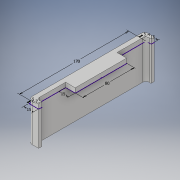
# Autodesk Inventor part: Part2
Saved by Autodesk Inventor 2018 (Build 220112000, 112)
## iProperties
Created: 2019-02-25
Part Number: Part2
Material: Generic
Document SubType Name: Modeling
Designer: ayoub
Density: 1 g/cm^3
Appearance: Default
Author: ayoub
Autodesk Inventor part; units mm, degrees
(part 1 of 2)
ref_plane "YZ Plane" through (0, 0, 0) normal (1, 0, 0) x (0, 1, 0)
ref_plane "XZ Plane" through (0, 0, 0) normal (0, 1, 0) x (-1, 0, 0)
ref_plane "XY Plane" through (0, 0, 0) normal (0, 0, 1) x (1, 0, 0)
sketch "Sketch1" plane through (0, 0, 0) normal (0, 1, 0) x (-1, 0, 0)
  line L0 (0, 40) -> (15, 40)
  line L1 (15, 40) -> (15, -40)
  line L2 (15, -40) -> (0, -40)
  line L3 (0, -40) -> (0, 40)
  line L4 (15, 85) -> (22, 85)
  line L5 (22, 85) -> (22, -85)
  line L6 (22, -85) -> (15, -85)
  line L7 (15, -85) -> (15, 85)
  line L8 (22, 85) -> (7, 85)
  line L9 (7, 85) -> (7, 90)
  line L10 (7, 90) -> (22, 90)
  line L11 (22, 90) -> (22, 85)
  line L12 (22, -85) -> (7, -85)
  line L13 (7, -85) -> (7, -90)
  line L14 (7, -90) -> (22, -90)
  line L15 (22, -90) -> (22, -85)
  point P0 (0, 0)
  point P1 (0, 0)
  point P2 (15, 0)
  dimension "d0" = 80
  dimension "d1" = 15
  dimension "d4" = 15
  dimension "d5" = 15
  dimension "d6" = 5
  dimension "d7" = 170
  dimension "d8" = 5
  dimension "d9" = 7
  constraints: 32 end point, 8 parallel, 4 horizontal, 4 perpendicular, 3 midpoint, 1 coincident
  measures "d0" distance of L2.end L0.start
  measures "d1" distance of L0.start L0.end
  measures "d4" distance of L9.end L10.end
  measures "d5" distance of L13.end L14.end
  measures "d6" distance of L10.end L4.end
  measures "d7" distance of L6.end L4.start
  measures "d8" distance of L14.end L5.end
  measures "d9" distance of L4.start L4.end
extrude "Extrusion1" add sketch "Sketch1" along normal blind 7 contours L0 L1 L2 L3
extrude "Extrusion2" add sketch "Sketch1" along normal blind 7 and the other way blind 53 contours L7 L4 L5 L6 L1
extrude "Extrusion3" add sketch "Sketch1" along normal blind 7 and the other way blind 53 contours L8 L9 L10 L11 L4 | L6 L15 L14 L13 L12
fillet "Fillet1" radius 5 1 edges at (-22, -23, 90)
fillet "Fillet2" radius 5 1 edges at (-22, -23, -90)
fillet "Fillet3" radius 5 1 edges at (-15, -23, -85)
fillet "Fillet4" radius 5 1 edges at (-15, -23, 85)
sketch "Sketch2" plane through (-22, -53, 85) normal (-1, 0, 0) x (0, 0, 1)
  line L0 (-170, 0) -> (-170, 60) projected
  line L1 (-18, 7.3167) -> (-152, 7.3167) construction
  line L2 (-152, 7.3167) -> (-152, 22.3167) construction
  line L3 (-152, 27.3167) -> (-18, 27.3167) construction
  line L4 (-18, 27.3167) -> (-18, 7.3167) construction
  line L5 (0, 60) -> (0, 0) projected
  line L6 (-147, 7.3167) -> (-142, 7.3167)
  line L7 (-142, 7.3167) -> (-142, 12.3167)
  line L8 (-142, 12.3167) -> (-146, 12.3167)
  line L9 (-147, 13.3167) -> (-147, 21.3167)
  line L10 (-146, 22.3167) -> (-142, 22.3167)
  line L11 (-142, 22.3167) -> (-142, 27.3167)
  line L12 (-142, 27.3167) -> (-147, 27.3167)
  line L13 (-28, 7.3167) -> (-23, 7.3167)
  line L14 (-23, 27.3167) -> (-28, 27.3167)
  line L15 (-28, 27.3167) -> (-28, 22.3167)
  line L16 (-28, 12.3167) -> (-28, 7.3167)
  line L17 (-18, 12.3167) -> (-18, 22.3167)
  arc A0 (-23, 7.3167) -> (-18, 12.3167) centre (-23, 12.3167) ccw
  arc A1 (-18, 22.3167) -> (-23, 27.3167) centre (-23, 22.3167) ccw
  arc A2 (-147, 27.3167) -> (-152, 22.3167) centre (-147, 22.3167) ccw
  arc A3 (-152, 12.3167) -> (-147, 7.3167) centre (-147, 12.3167) ccw
  arc A4 (-147, 13.3167) -> (-146, 12.3167) centre (-146, 13.3167) ccw
  arc A5 (-146, 22.3167) -> (-147, 21.3167) centre (-146, 21.3167) ccw
  line L18 (-51.6825, 53.4391) -> (-114.3216, 53.4391) construction
  line L19 (-114.3216, 53.4391) -> (-114.3216, 31.9963) construction
  line L20 (-114.3216, 31.9963) -> (-51.6825, 31.9963) construction
  line L21 (-51.6825, 31.9963) -> (-51.6825, 53.4391) construction
  line L22 (-152, 12.3167) -> (-152, 22.3167)
  line L23 (-24, 12.3167) -> (-28, 12.3167)
  line L24 (-24, 22.3167) -> (-28, 22.3167)
  line L25 (-23, 13.3167) -> (-23, 21.3167)
  arc A6 (-24, 12.3167) -> (-23, 13.3167) centre (-24, 13.3167) ccw
  arc A7 (-23, 21.3167) -> (-24, 22.3167) centre (-24, 21.3167) ccw
  line L26 (-147.3155, 50.9956) -> (-166.2914, 50.9956) construction
  line L27 (-166.2914, 50.9956) -> (-166.2914, 58.7345) construction
  line L28 (-166.2914, 58.7345) -> (-147.3155, 58.7345) construction
  line L29 (-147.3155, 58.7345) -> (-147.3155, 50.9956) construction
  line L30 (-48.6554, 17.8276) -> (-37.2597, 17.8276)
  spline S0 degree 2 poles (-37.2597, 17.8276) (-37.3507, 18.212) (-39.1918, 18.6925) (-40.4209, 18.6925) knots 0 0 0 1 2 2 2
  spline S1 degree 2 poles (-40.4209, 18.6925) (-42.6111, 18.6925) (-43.8553, 18.1968) knots 0 0 0 1 1 1
  line L31 (-43.8553, 18.1968) -> (-48.2255, 18.561)
  spline S2 degree 2 poles (-48.2255, 18.561) (-45.7926, 19.6232) (-40.6637, 19.6232) knots 0 0 0 1 1 1
  spline S3 degree 2 poles (-40.6637, 19.6232) (-36.8904, 19.6232) (-32.4292, 18.4801) (-32.4292, 17.514) knots 0 0 0 1 2 2 2
  spline S4 degree 2 poles (-32.4292, 17.514) (-32.4292, 16.644) (-37.1332, 15.4655) (-40.5727, 15.4655) knots 0 0 0 1 2 2 2
  spline S5 degree 2 poles (-40.5727, 15.4655) (-44.0273, 15.4655) (-48.6554, 16.7047) (-48.6554, 17.6354) knots 0 0 0 1 2 2 2
  line L32 (-48.6554, 17.6354) -> (-48.6554, 17.8276)
  line L33 (-37.2951, 17.0284) -> (-43.7289, 17.0284)
  spline S6 degree 2 poles (-43.7289, 17.0284) (-43.0612, 16.2798) (-40.6587, 16.2798) knots 0 0 0 1 1 1
  spline S7 degree 2 poles (-40.6587, 16.2798) (-39.2829, 16.2798) (-37.4822, 16.6693) (-37.2951, 17.0284) knots 0 0 0 1 2 2 2
  line L34 (-50.7393, 15.5414) -> (-56.5763, 15.5414)
  line L35 (-56.5763, 15.5414) -> (-59.8084, 16.5378)
  line L36 (-59.8084, 16.5378) -> (-63.0051, 15.5414)
  line L37 (-63.0051, 15.5414) -> (-68.8269, 15.5414)
  line L38 (-68.8269, 15.5414) -> (-62.7117, 17.4533)
  line L39 (-62.7117, 17.4533) -> (-69.4035, 19.5372)
  line L40 (-69.4035, 19.5372) -> (-63.5311, 19.5372)
  line L41 (-63.5311, 19.5372) -> (-59.8034, 18.3587)
  line L42 (-59.8034, 18.3587) -> (-56.0402, 19.5372)
  line L43 (-56.0402, 19.5372) -> (-50.183, 19.5372)
  line L44 (-50.183, 19.5372) -> (-56.8495, 17.4482)
  line L45 (-56.8495, 17.4482) -> (-50.7393, 15.5414)
  line L46 (-77.0715, 15.5515) -> (-77.0715, 16.1332)
  line L47 (-77.0715, 16.1332) -> (-77.1474, 16.1332)
  spline S8 degree 2 poles (-77.1474, 16.1332) (-78.1893, 15.7841) (-80.4351, 15.4655) (-82.0183, 15.4655) knots 0 0 0 1 2 2 2
  spline S9 degree 2 poles (-82.0183, 15.4655) (-84.8811, 15.4655) (-88.9175, 16.7199) (-88.9175, 17.6152) knots 0 0 0 1 2 2 2
  spline S10 degree 2 poles (-88.9175, 17.6152) (-88.9175, 18.4396) (-84.9924, 19.6131) (-82.2965, 19.6131) knots 0 0 0 1 2 2 2
  spline S11 degree 2 poles (-82.2965, 19.6131) (-80.6425, 19.6131) (-78.4119, 19.2691) (-77.2233, 18.8948) knots 0 0 0 1 2 2 2
  line L48 (-77.2233, 18.8948) -> (-77.1474, 18.8948)
  line L49 (-77.1474, 18.8948) -> (-77.1474, 21.2974)
  line L50 (-77.1474, 21.2974) -> (-72.317, 21.2974)
  line L51 (-72.317, 21.2974) -> (-72.317, 15.5515)
  line L52 (-72.317, 15.5515) -> (-77.0715, 15.5515)
  spline S12 degree 2 poles (-83.9353, 17.605) (-83.9353, 17.2156) (-81.9272, 16.6541) (-80.5312, 16.6541) knots 0 0 0 1 2 2 2
  spline S13 degree 2 poles (-80.5312, 16.6541) (-79.1554, 16.6541) (-77.2233, 17.2055) (-77.2233, 17.605) knots 0 0 0 1 2 2 2
  spline S14 degree 2 poles (-77.2233, 17.605) (-77.2233, 17.9945) (-79.2515, 18.5408) (-80.6981, 18.5408) knots 0 0 0 1 2 2 2
  spline S15 degree 2 poles (-80.6981, 18.5408) (-82.1144, 18.5408) (-83.9353, 18.0198) (-83.9353, 17.605) knots 0 0 0 1 2 2 2
  line L53 (-92.6301, 13.3361) -> (-97.3897, 13.3361)
  line L54 (-97.3897, 13.3361) -> (-97.3897, 19.5372)
  line L55 (-97.3897, 19.5372) -> (-92.6301, 19.5372)
  line L56 (-92.6301, 19.5372) -> (-92.6301, 13.3361)
  line L57 (-117.1818, 17.8276) -> (-105.786, 17.8276)
  spline S16 degree 2 poles (-105.786, 17.8276) (-105.8771, 18.212) (-107.7182, 18.6925) (-108.9473, 18.6925) knots 0 0 0 1 2 2 2
  spline S17 degree 2 poles (-108.9473, 18.6925) (-111.1374, 18.6925) (-112.3817, 18.1968) knots 0 0 0 1 1 1
  line L58 (-112.3817, 18.1968) -> (-116.7519, 18.561)
  spline S18 degree 2 poles (-116.7519, 18.561) (-114.3189, 19.6232) (-109.1901, 19.6232) knots 0 0 0 1 1 1
  spline S19 degree 2 poles (-109.1901, 19.6232) (-105.4168, 19.6232) (-100.9556, 18.4801) (-100.9556, 17.514) knots 0 0 0 1 2 2 2
  spline S20 degree 2 poles (-100.9556, 17.514) (-100.9556, 16.644) (-105.6596, 15.4655) (-109.099, 15.4655) knots 0 0 0 1 2 2 2
  spline S21 degree 2 poles (-109.099, 15.4655) (-112.5537, 15.4655) (-117.1818, 16.7047) (-117.1818, 17.6354) knots 0 0 0 1 2 2 2
  line L59 (-117.1818, 17.6354) -> (-117.1818, 17.8276)
  line L60 (-105.8214, 17.0284) -> (-112.2553, 17.0284)
  spline S22 degree 2 poles (-112.2553, 17.0284) (-111.5876, 16.2798) (-109.185, 16.2798) knots 0 0 0 1 1 1
  spline S23 degree 2 poles (-109.185, 16.2798) (-107.8092, 16.2798) (-106.0086, 16.6693) (-105.8214, 17.0284) knots 0 0 0 1 2 2 2
  spline S24 degree 2 poles (-120.1003, 17.5494) (-120.1003, 16.6238) (-124.8245, 15.4554) (-128.5219, 15.4554) knots 0 0 0 1 2 2 2
  spline S25 degree 2 poles (-128.5219, 15.4554) (-131.9614, 15.4554) (-136.63, 16.6491) (-136.63, 17.5342) knots 0 0 0 1 2 2 2
  spline S26 degree 2 poles (-136.63, 17.5342) (-136.63, 18.4346) (-131.9614, 19.6232) (-128.4511, 19.6232) knots 0 0 0 1 2 2 2
  spline S27 degree 2 poles (-128.4511, 19.6232) (-124.4907, 19.6232) (-120.1003, 18.3637) (-120.1003, 17.5494) knots 0 0 0 1 2 2 2
  spline S28 degree 2 poles (-131.9462, 17.5494) (-131.9462, 17.1448) (-129.8269, 16.5429) (-128.4107, 16.5429) knots 0 0 0 1 2 2 2
  spline S29 degree 2 poles (-128.4107, 16.5429) (-126.9388, 16.5429) (-124.8194, 17.1094) (-124.8194, 17.5039) knots 0 0 0 1 2 2 2
  spline S30 degree 2 poles (-124.8194, 17.5039) (-124.8194, 17.9389) (-126.9236, 18.5408) (-128.4107, 18.5408) knots 0 0 0 1 2 2 2
  spline S31 degree 2 poles (-128.4107, 18.5408) (-129.8269, 18.5408) (-131.9462, 17.949) (-131.9462, 17.5494) knots 0 0 0 1 2 2 2
  spline S32 degree 2 poles (-57.495, 42.9117) (-57.495, 43.0373) (-57.1013, 43.3568) (-56.4394, 43.7049) (-55.5606, 44.0758) (-55.0699, 44.2641) knots 0 0 0 1 2 3 4 4 4
  spline S33 degree 2 poles (-55.0699, 44.2641) (-54.408, 44.5152) (-52.9129, 44.9774) (-51.3722, 45.3369) (-49.8429, 45.548) (-49.1525, 45.548) knots 0 0 0 1 2 3 4 4 4
  spline S34 degree 2 poles (-49.1525, 45.548) (-48.3251, 45.548) (-47.1153, 45.3141) (-46.3222, 44.8804) (-45.9399, 44.2755) (-45.9399, 43.8989) knots 0 0 0 1 2 3 4 4 4
  spline S35 degree 2 poles (-45.9399, 43.8989) (-45.9399, 43.5908) (-46.2252, 42.946) (-46.7387, 42.3069) (-47.4292, 41.7191) (-47.8286, 41.468) knots 0 0 0 1 2 3 4 4 4
  spline S36 degree 2 poles (-47.8286, 41.468) (-48.0569, 41.3254) (-48.6903, 41.0115) (-49.3979, 40.7091) (-50.1168, 40.4466) (-50.4421, 40.3496) knots 0 0 0 1 2 3 4 4 4
  spline S37 degree 2 poles (-50.4421, 40.3496) (-50.6761, 40.2811) (-51.3779, 40.1099) (-52.154, 39.9616) (-52.9015, 39.8646) (-53.1754, 39.8646) knots 0 0 0 1 2 3 4 4 4
  spline S38 degree 2 poles (-53.1754, 39.8646) (-53.6661, 39.8646) (-54.2425, 39.9273) (-54.465, 40.0129) knots 0 0 0 1 2 2 2
  spline S39 degree 2 poles (-54.465, 40.0129) (-54.5734, 40.0529) (-54.8473, 40.2184) (-55.0927, 40.4124) (-55.2639, 40.6007) (-55.2639, 40.6692) knots 0 0 0 1 2 3 4 4 4
  spline S40 degree 2 poles (-55.2639, 40.6692) (-55.2639, 40.7091) (-55.1555, 40.8575) (-54.9843, 41.0287) (-54.7675, 41.217) (-54.5563, 41.3824) (-54.3737, 41.508) (-54.3224, 41.5422) knots 0 0 0 1 2 3 4 5 6 6 6
  spline S41 degree 2 poles (-54.3224, 41.5422) (-53.9971, 41.7305) (-53.5064, 41.7305) knots 0 0 0 1 1 1
  spline S42 degree 2 poles (-53.5064, 41.7305) (-53.0955, 41.7305) (-52.639, 41.5023) (-52.639, 41.3311) knots 0 0 0 1 2 2 2
  spline S43 degree 2 poles (-52.639, 41.3311) (-52.639, 41.274) (-52.8844, 41.0401) (-53.1697, 40.9031) knots 0 0 0 1 2 2 2
  spline S44 degree 2 poles (-53.1697, 40.9031) (-53.3066, 40.8346) (-53.5064, 40.6977) (-53.5634, 40.6463) knots 0 0 0 1 2 2 2
  spline S45 degree 2 poles (-53.5634, 40.6463) (-53.3865, 40.6178) (-53.1982, 40.6178) knots 0 0 0 1 1 1
  spline S46 degree 2 poles (-53.1982, 40.6178) (-52.9757, 40.6178) (-52.3023, 40.7262) (-51.5719, 40.8974) (-50.8815, 41.1085) (-50.6475, 41.2056) knots 0 0 0 1 2 3 4 4 4
  spline S47 degree 2 poles (-50.6475, 41.2056) (-49.9799, 41.4737) (-48.7987, 42.1528) (-48.4107, 42.5522) knots 0 0 0 1 2 2 2
  spline S48 degree 2 poles (-48.4107, 42.5522) (-48.2566, 42.712) (-47.9827, 43.0715) (-47.783, 43.4424) (-47.6689, 43.8133) (-47.6689, 43.9788) knots 0 0 0 1 2 3 4 4 4
  spline S49 degree 2 poles (-47.6689, 43.9788) (-47.6689, 44.1614) (-47.8286, 44.4695) (-48.1938, 44.7035) (-48.7873, 44.829) (-49.2153, 44.829) knots 0 0 0 1 2 3 4 4 4
  spline S50 degree 2 poles (-49.2153, 44.829) (-49.7288, 44.829) (-50.853, 44.6921) (-52.0056, 44.4467) (-53.1697, 44.1386) (-54.2425, 43.7905) (-55.2011, 43.4367) (-55.5892, 43.2769) knots 0 0 0 1 2 3 4 5 6 6 6
  spline S51 degree 2 poles (-55.5892, 43.2769) (-55.7432, 43.2199) (-56.1084, 43.0544) (-56.4907, 42.8718) (-56.8559, 42.6835) (-57.01, 42.6036) knots 0 0 0 1 2 3 4 4 4
  spline S52 degree 2 poles (-57.01, 42.6036) (-57.1755, 42.6492) (-57.3695, 42.712) (-57.4608, 42.7805) (-57.495, 42.8604) (-57.495, 42.9117) knots 0 0 0 1 2 3 4 4 4
  spline S53 degree 2 poles (-67.9832, 44.9146) (-67.9832, 45.0059) (-67.8462, 45.16) (-67.6066, 45.2798) (-67.2699, 45.354) (-67.0759, 45.354) knots 0 0 0 1 2 3 4 4 4
  spline S54 degree 2 poles (-67.0759, 45.354) (-66.8933, 45.354) (-66.5509, 45.2399) (-66.2256, 45.0573) (-65.9289, 44.829) (-65.6892, 44.6008) (-65.5066, 44.3896) (-65.4439, 44.3212) knots 0 0 0 1 2 3 4 5 6 6 6
  spline S55 degree 2 poles (-65.4439, 44.3212) (-65.3697, 44.2242) (-65.2099, 44.0587) (-65.1243, 43.9331) knots 0 0 0 1 2 2 2
  spline S56 degree 2 poles (-65.1243, 43.9331) (-65.073, 43.859) (-65.0216, 43.7848) (-64.9874, 43.7448) (-64.9646, 43.722) (-64.9474, 43.6992) knots 0 0 0 1 2 3 4 4 4
  spline S57 degree 2 poles (-64.9474, 43.6992) (-64.8048, 43.7277) (-64.4738, 43.7391) (-64.2741, 43.7391) knots 0 0 0 1 2 2 2
  spline S58 degree 2 poles (-64.2741, 43.7391) (-64.2341, 43.7391) (-64.063, 43.7677) (-63.8404, 43.8019) (-63.6008, 43.8418) (-63.4923, 43.8533) knots 0 0 0 1 2 3 4 4 4
  spline S59 degree 2 poles (-63.4923, 43.8533) (-63.1443, 43.8989) (-62.3397, 43.9788) (-61.4609, 44.053) (-60.5422, 44.1272) (-60.0857, 44.1671) knots 0 0 0 1 2 3 4 4 4
  spline S60 degree 2 poles (-60.0857, 44.1671) (-60.0343, 44.1728) (-59.9602, 44.1956) (-59.8289, 44.2812) (-59.5721, 44.4695) (-59.3325, 44.6464) knots 0 0 0 1 2 3 4 4 4
  spline S61 degree 2 poles (-59.3325, 44.6464) (-59.0586, 44.8404) (-58.5678, 45.1315) (-58.351, 45.2399) knots 0 0 0 1 2 2 2
  spline S62 degree 2 poles (-58.351, 45.2399) (-58.1456, 45.3426) (-57.6776, 45.451) (-57.4209, 45.451) knots 0 0 0 1 2 2 2
  spline S63 degree 2 poles (-57.4209, 45.451) (-57.0899, 45.451) (-56.5706, 45.3654) (-56.2225, 45.2399) (-56.0399, 45.0858) (-56.0399, 45.023) knots 0 0 0 1 2 3 4 4 4
  spline S64 degree 2 poles (-56.0399, 45.023) (-56.0399, 44.8975) (-56.4565, 44.8005) (-56.8274, 44.772) knots 0 0 0 1 2 2 2
  spline S65 degree 2 poles (-56.8274, 44.772) (-56.8274, 44.7663) (-56.9815, 44.6635) (-57.1983, 44.538) (-57.4095, 44.4125) (-57.4551, 44.3782) knots 0 0 0 1 2 3 4 4 4
  spline S66 degree 2 poles (-57.4551, 44.3782) (-57.7347, 44.1842) (-58.3453, 43.762) (-58.7162, 43.4881) knots 0 0 0 1 2 2 2
  line L61 (-58.7162, 43.4881) -> (-58.7162, 43.4938)
  spline S67 degree 2 poles (-58.7162, 43.4938) (-58.8988, 43.3568) (-59.1385, 43.1742) (-59.3553, 43.0144) (-59.595, 42.849) (-59.7661, 42.7291) knots 0 0 0 1 2 3 4 4 4
  spline S68 degree 2 poles (-59.7661, 42.7291) (-60.2112, 42.4153) (-60.8846, 41.9759) (-61.1014, 41.8332) knots 0 0 0 1 2 2 2
  spline S69 degree 2 poles (-61.1014, 41.8332) (-61.3582, 41.6335) (-61.5921, 41.4509) knots 0 0 0 1 1 1
  spline S70 degree 2 poles (-61.5921, 41.4509) (-61.6892, 41.371) (-61.8775, 41.2056) (-62.0486, 41.0572) (-62.1856, 40.9202) (-62.2255, 40.8746) knots 0 0 0 1 2 3 4 4 4
  spline S71 degree 2 poles (-62.2255, 40.8746) (-63.0815, 39.8246) (-63.6921, 39.8246) knots 0 0 0 1 1 1
  spline S72 degree 2 poles (-63.6921, 39.8246) (-63.9602, 39.8246) (-64.2912, 39.8646) (-64.4738, 39.9616) (-64.5366, 40.1214) (-64.5366, 40.2412) knots 0 0 0 1 2 3 4 4 4
  spline S73 degree 2 poles (-64.5366, 40.2412) (-64.5366, 40.3553) (-64.5366, 40.4809) (-64.5252, 40.5722) (-64.5138, 40.6692) (-64.5023, 40.7433) knots 0 0 0 1 2 3 4 4 4
  spline S74 degree 2 poles (-64.5023, 40.7433) (-64.6735, 40.9316) (-64.9988, 41.3197) (-65.1414, 41.508) knots 0 0 0 1 2 2 2
  spline S75 degree 2 poles (-65.1414, 41.508) (-65.17, 41.5536) (-65.3697, 41.8275) (-65.6322, 42.2041) (-65.9289, 42.6207) (-66.18, 42.9916) (-66.3683, 43.2541) (-66.3968, 43.294) knots 0 0 0 1 2 3 4 5 6 6 6
  spline S76 degree 2 poles (-66.3968, 43.294) (-66.4938, 43.4938) (-66.9218, 43.9617) knots 0 0 0 1 1 1
  spline S77 degree 2 poles (-66.9218, 43.9617) (-66.9789, 44.0187) (-67.0588, 44.1043) (-67.1672, 44.1956) (-67.3441, 44.3212) (-67.4867, 44.4182) knots 0 0 0 1 2 3 4 4 4
  spline S78 degree 2 poles (-67.4867, 44.4182) (-67.9832, 44.7548) (-67.9832, 44.9146) knots 0 0 0 1 1 1
  spline S79 degree 2 poles (-63.1671, 43.1) (-63.4866, 43.0601) (-64.1428, 42.9745) (-64.4225, 42.9288) knots 0 0 0 1 2 2 2
  spline S80 degree 2 poles (-64.4225, 42.9288) (-64.3083, 42.7519) (-64.063, 42.3696) (-63.7948, 41.993) (-63.5209, 41.6335) (-63.3725, 41.4852) knots 0 0 0 1 2 3 4 4 4
  spline S81 degree 2 poles (-63.3725, 41.4852) (-62.7562, 41.9074) (-61.5237, 42.8261) (-60.9702, 43.3055) knots 0 0 0 1 2 2 2
  spline S82 degree 2 poles (-60.9702, 43.3055) (-61.187, 43.294) (-61.6606, 43.2883) (-61.809, 43.2655) knots 0 0 0 1 2 2 2
  spline S83 degree 2 poles (-61.809, 43.2655) (-62.003, 43.237) (-62.3111, 43.1913) (-62.6193, 43.1571) (-62.9502, 43.1171) (-63.1671, 43.1) knots 0 0 0 1 2 3 4 4 4
  spline S84 degree 2 poles (-81.4842, 45.023) (-81.4785, 45.12) (-81.2445, 45.2684) (-81.0391, 45.3255) knots 0 0 0 1 2 2 2
  spline S85 degree 2 poles (-81.0391, 45.3255) (-80.8907, 45.3654) (-80.5255, 45.4054) (-80.3372, 45.4054) knots 0 0 0 1 2 2 2
  spline S86 degree 2 poles (-80.3372, 45.4054) (-79.9036, 45.4054) (-79.0704, 45.2285) (-78.5854, 45.0687) knots 0 0 0 1 2 2 2
  spline S87 degree 2 poles (-78.5854, 45.0687) (-78.3457, 44.9888) (-77.6153, 44.7263) (-77.136, 44.5437) knots 0 0 0 1 2 2 2
  spline S88 degree 2 poles (-77.136, 44.5437) (-77.0219, 44.4981) (-76.3428, 44.2356) (-75.7836, 44.013) knots 0 0 0 1 2 2 2
  spline S89 degree 2 poles (-75.7836, 44.013) (-75.2644, 43.8076) (-74.6424, 43.5737) (-74.6024, 43.5622) knots 0 0 0 1 2 2 2
  spline S90 degree 2 poles (-74.6024, 43.5622) (-74.5111, 43.5451) (-74.3457, 43.5394) (-74.1231, 43.5394) knots 0 0 0 1 2 2 2
  spline S91 degree 2 poles (-74.1231, 43.5394) (-74.0718, 43.5394) (-73.9747, 43.5394) (-73.8378, 43.5451) (-73.6153, 43.5508) (-73.4269, 43.5622) knots 0 0 0 1 2 3 4 4 4
  spline S92 degree 2 poles (-73.4269, 43.5622) (-72.9876, 43.4025) (-72.9876, 43.14) knots 0 0 0 1 1 1
  spline S93 degree 2 poles (-72.9876, 43.14) (-72.9876, 43.0087) (-73.2329, 42.8432) (-73.4612, 42.8033) knots 0 0 0 1 2 2 2
  spline S94 degree 2 poles (-73.4612, 42.8033) (-73.5182, 42.7976) (-73.5753, 42.7862) (-73.6438, 42.7862) (-73.7579, 42.7748) (-73.8663, 42.7691) knots 0 0 0 1 2 3 4 4 4
  spline S95 degree 2 poles (-73.8663, 42.7691) (-74.0718, 42.7691) (-74.4655, 42.7177) (-74.8307, 42.6435) (-75.1674, 42.5522) (-75.3271, 42.5123) knots 0 0 0 1 2 3 4 4 4
  spline S96 degree 2 poles (-75.3271, 42.5123) (-75.5611, 42.4552) (-76.0575, 42.3069) (-76.3086, 42.2213) knots 0 0 0 1 2 2 2
  spline S97 degree 2 poles (-76.3086, 42.2213) (-76.5312, 42.1471) (-76.9591, 41.9645) (-77.1646, 41.8618) knots 0 0 0 1 2 2 2
  spline S98 degree 2 poles (-77.1646, 41.8618) (-77.33, 41.7819) (-77.4841, 41.6107) (-77.4841, 41.5251) knots 0 0 0 1 2 2 2
  spline S99 degree 2 poles (-77.4841, 41.5251) (-77.4841, 41.3996) (-77.1646, 41.1713) (-76.6852, 40.983) (-76.1146, 40.8461) (-75.8635, 40.8118) knots 0 0 0 1 2 3 4 4 4
  spline S100 degree 2 poles (-75.8635, 40.8118) (-75.3614, 40.7376) (-74.882, 40.7376) knots 0 0 0 1 1 1
  spline S101 degree 2 poles (-74.882, 40.7376) (-74.7394, 40.7376) (-74.3057, 40.7548) (-74.0375, 40.7662) knots 0 0 0 1 2 2 2
  spline S102 degree 2 poles (-74.0375, 40.7662) (-73.7921, 40.7833) (-73.3242, 40.8061) (-73.1074, 40.8232) knots 0 0 0 1 2 2 2
  spline S103 degree 2 poles (-73.1074, 40.8232) (-73.0047, 40.8346) (-72.8906, 40.8403) (-72.7764, 40.8518) (-72.6224, 40.8632) (-72.4968, 40.8803) knots 0 0 0 1 2 3 4 4 4
  spline S104 degree 2 poles (-72.4968, 40.8803) (-72.5539, 40.9488) (-72.6395, 41.0971) (-72.6737, 41.1884) knots 0 0 0 1 2 2 2
  spline S105 degree 2 poles (-72.6737, 41.1884) (-72.7422, 41.3311) (-72.7764, 41.565) (-72.7764, 41.6563) knots 0 0 0 1 2 2 2
  spline S106 degree 2 poles (-72.7764, 41.6563) (-72.7764, 41.7648) (-72.7707, 41.9588) (-72.7536, 42.0558) knots 0 0 0 1 2 2 2
  spline S107 degree 2 poles (-72.7536, 42.0558) (-72.7308, 42.2441) (-72.668, 42.4381) knots 0 0 0 1 1 1
  spline S108 degree 2 poles (-72.668, 42.4381) (-72.6052, 42.6207) (-72.4968, 42.9231) knots 0 0 0 1 1 1
  spline S109 degree 2 poles (-72.4968, 42.9231) (-72.4112, 43.1799) (-72.2914, 43.5679) (-72.2572, 43.722) knots 0 0 0 1 2 2 2
  spline S110 degree 2 poles (-72.2572, 43.722) (-72.2229, 43.8647) (-72.183, 44.1386) (-72.183, 44.2641) knots 0 0 0 1 2 2 2
  spline S111 degree 2 poles (-72.183, 44.2641) (-72.183, 44.3725) (-72.2286, 44.578) (-72.3199, 44.7663) (-72.4854, 44.9546) (-72.6109, 45.0573) knots 0 0 0 1 2 3 4 4 4
  spline S112 degree 2 poles (-72.6109, 45.0573) (-72.5368, 45.1143) (-72.3142, 45.2114) (-72.0631, 45.2912) (-71.8007, 45.3369) (-71.6865, 45.3369) knots 0 0 0 1 2 3 4 4 4
  spline S113 degree 2 poles (-71.6865, 45.3369) (-71.1045, 45.3369) (-70.8363, 45.2171) knots 0 0 0 1 1 1
  spline S114 degree 2 poles (-70.8363, 45.2171) (-70.5339, 45.0858) (-70.4711, 44.9146) knots 0 0 0 1 1 1
  spline S115 degree 2 poles (-70.4711, 44.9146) (-70.4312, 44.829) (-70.414, 44.6122) (-70.414, 44.4752) knots 0 0 0 1 2 2 2
  spline S116 degree 2 poles (-70.414, 44.4752) (-70.414, 44.2755) (-70.454, 44.0929) knots 0 0 0 1 1 1
  spline S117 degree 2 poles (-70.454, 44.0929) (-70.4939, 43.9331) (-70.5852, 43.6307) (-70.6423, 43.4824) knots 0 0 0 1 2 2 2
  spline S118 degree 2 poles (-70.6423, 43.4824) (-70.6765, 43.4196) (-70.7222, 43.3055) (-70.7564, 43.1799) (-70.8021, 43.0316) (-70.8306, 42.9345) knots 0 0 0 1 2 3 4 4 4
  spline S119 degree 2 poles (-70.8306, 42.9345) (-70.9219, 42.6378) (-71.0417, 42.09) (-71.0417, 41.8618) knots 0 0 0 1 2 2 2
  spline S120 degree 2 poles (-71.0417, 41.8618) (-71.0417, 41.6906) (-71.0018, 41.314) (-70.9618, 41.1085) knots 0 0 0 1 2 2 2
  spline S121 degree 2 poles (-70.9618, 41.1085) (-70.7279, 41.1371) (-70.414, 41.1713) (-70.357, 41.1713) knots 0 0 0 1 2 2 2
  spline S122 degree 2 poles (-70.357, 41.1713) (-69.9747, 41.1713) (-69.7179, 40.9887) (-69.7179, 40.8232) knots 0 0 0 1 2 2 2
  spline S123 degree 2 poles (-69.7179, 40.8232) (-69.7179, 40.6349) (-70.3684, 40.4751) knots 0 0 0 1 1 1
  spline S124 degree 2 poles (-70.3684, 40.4751) (-70.6195, 40.4124) (-71.133, 40.3154) (-71.3841, 40.2754) knots 0 0 0 1 2 2 2
  spline S125 degree 2 poles (-71.3841, 40.2754) (-71.6637, 40.2298) (-72.4455, 40.1499) (-72.9134, 40.1157) knots 0 0 0 1 2 2 2
  spline S126 degree 2 poles (-72.9134, 40.1157) (-73.3585, 40.0814) (-74.1688, 40.0415) (-74.4826, 40.0415) knots 0 0 0 1 2 2 2
  spline S127 degree 2 poles (-74.4826, 40.0415) (-75.5782, 40.0415) (-76.5939, 40.1727) knots 0 0 0 1 1 1
  spline S128 degree 2 poles (-76.5939, 40.1727) (-77.1303, 40.2412) (-78.0262, 40.4694) (-78.3743, 40.6349) knots 0 0 0 1 2 2 2
  spline S129 degree 2 poles (-78.3743, 40.6349) (-79.156, 40.983) (-79.156, 41.5365) knots 0 0 0 1 1 1
  spline S130 degree 2 poles (-79.156, 41.5365) (-79.156, 41.896) (-78.6025, 42.2498) knots 0 0 0 1 1 1
  spline S131 degree 2 poles (-78.6025, 42.2498) (-78.1346, 42.5351) (-76.9192, 42.9631) (-76.1945, 43.1628) knots 0 0 0 1 2 2 2
  spline S132 degree 2 poles (-76.1945, 43.1628) (-76.4227, 43.2484) (-76.8849, 43.4139) (-77.1531, 43.4995) knots 0 0 0 1 2 2 2
  spline S133 degree 2 poles (-77.1531, 43.4995) (-77.5469, 43.6364) (-78.2316, 43.8818) (-78.5341, 43.9902) knots 0 0 0 1 2 2 2
  spline S134 degree 2 poles (-78.5341, 43.9902) (-78.8365, 44.0929) (-79.5669, 44.344) (-80.0063, 44.4981) knots 0 0 0 1 2 2 2
  spline S135 degree 2 poles (-80.0063, 44.4981) (-80.4228, 44.635) (-81.1247, 44.8633) (-81.353, 44.9374) knots 0 0 0 1 2 2 2
  line L62 (-81.353, 44.9374) -> (-81.4842, 45.023)
  spline S136 degree 2 poles (-92.6114, 40.2241) (-92.6114, 40.2583) (-92.5315, 40.3781) (-92.3946, 40.5037) (-92.2234, 40.6064) (-92.1264, 40.6292) knots 0 0 0 1 2 3 4 4 4
  spline S137 degree 2 poles (-92.1264, 40.6292) (-91.9438, 40.6749) (-91.59, 40.7148) (-91.3389, 40.7433) knots 0 0 0 1 2 2 2
  spline S138 degree 2 poles (-91.3389, 40.7433) (-90.6713, 40.8061) (-89.4045, 40.8917) (-88.2747, 40.9488) (-87.3331, 40.9716) (-87.0136, 40.9716) knots 0 0 0 1 2 3 4 4 4
  line L63 (-87.0136, 40.9716) -> (-85.9465, 40.9716)
  spline S139 degree 2 poles (-85.9465, 40.9716) (-85.7125, 40.9716) (-85.3245, 40.9716) (-85.1419, 40.9602) knots 0 0 0 1 2 2 2
  spline S140 degree 2 poles (-85.1419, 40.9602) (-85.1248, 41.08) (-85.0849, 41.4224) (-85.0449, 41.7705) (-84.9993, 42.1014) (-84.965, 42.2099) knots 0 0 0 1 2 3 4 4 4
  spline S141 degree 2 poles (-84.965, 42.2099) (-85.159, 42.2213) (-85.684, 42.2327) (-85.9294, 42.2327) knots 0 0 0 1 2 2 2
  spline S142 degree 2 poles (-85.9294, 42.2327) (-86.2832, 42.2327) (-86.985, 42.2041) (-87.2133, 42.1927) knots 0 0 0 1 2 2 2
  spline S143 degree 2 poles (-87.2133, 42.1927) (-87.3274, 42.187) (-87.8182, 42.1699) (-88.3717, 42.1528) (-88.9023, 42.1243) (-89.0507, 42.1014) knots 0 0 0 1 2 3 4 4 4
  spline S144 degree 2 poles (-89.0507, 42.1014) (-89.1934, 42.0729) (-89.4501, 42.0215) (-89.6841, 41.9873) (-89.9352, 41.9759) (-90.0835, 41.9759) knots 0 0 0 1 2 3 4 4 4
  spline S145 degree 2 poles (-90.0835, 41.9759) (-90.2776, 41.9759) (-90.5343, 42.0501) (-90.6827, 42.1756) (-90.7398, 42.3354) (-90.7398, 42.4267) knots 0 0 0 1 2 3 4 4 4
  spline S146 degree 2 poles (-90.7398, 42.4267) (-90.7398, 42.5351) (-90.5001, 42.6721) (-90.152, 42.7577) (-89.7697, 42.809) (-89.6327, 42.8204) knots 0 0 0 1 2 3 4 4 4
  spline S147 degree 2 poles (-89.6327, 42.8204) (-89.5129, 42.8375) (-88.8852, 42.8661) (-88.0635, 42.8946) (-87.1505, 42.9231) (-86.3288, 42.946) (-85.684, 42.9574) (-85.5471, 42.9574) knots 0 0 0 1 2 3 4 5 6 6 6
  spline S148 degree 2 poles (-85.5471, 42.9574) (-85.3245, 42.9574) (-84.9479, 42.9916) (-84.7425, 43.0201) knots 0 0 0 1 2 2 2
  spline S149 degree 2 poles (-84.7425, 43.0201) (-84.6569, 43.197) (-84.5542, 43.5965) (-84.4515, 43.819) knots 0 0 0 1 2 2 2
  spline S150 degree 2 poles (-84.4515, 43.819) (-84.4172, 43.9046) (-84.3373, 44.0872) (-84.2746, 44.247) (-84.2289, 44.3839) (-84.2232, 44.4296) knots 0 0 0 1 2 3 4 4 4
  spline S151 degree 2 poles (-84.2232, 44.4296) (-84.3716, 44.4296) (-84.771, 44.4182) (-85.2047, 44.4068) (-85.6441, 44.3896) (-85.8381, 44.3782) knots 0 0 0 1 2 3 4 4 4
  spline S152 degree 2 poles (-85.8381, 44.3782) (-86.3459, 44.3554) (-87.0763, 44.3212) (-87.6584, 44.2983) (-88.1548, 44.2698) (-88.4458, 44.247) knots 0 0 0 1 2 3 4 4 4
  spline S153 degree 2 poles (-88.4458, 44.247) (-88.5999, 44.2356) (-89.0222, 44.2128) (-89.4787, 44.1899) (-89.9295, 44.1557) (-90.1178, 44.1329) knots 0 0 0 1 2 3 4 4 4
  spline S154 degree 2 poles (-90.1178, 44.1329) (-90.2319, 44.1157) (-90.4716, 44.0701) (-90.7169, 44.0302) (-90.968, 44.0016) (-91.0993, 44.0016) knots 0 0 0 1 2 3 4 4 4
  spline S155 degree 2 poles (-91.0993, 44.0016) (-91.2476, 44.0016) (-91.5329, 44.0644) (-91.7498, 44.1785) (-91.8753, 44.344) (-91.8753, 44.4353) knots 0 0 0 1 2 3 4 4 4
  spline S156 degree 2 poles (-91.8753, 44.4353) (-91.8753, 44.4695) (-91.7384, 44.5837) (-91.5044, 44.7035) (-91.1677, 44.8062) (-90.9737, 44.8233) knots 0 0 0 1 2 3 4 4 4
  spline S157 degree 2 poles (-90.9737, 44.8233) (-90.3403, 44.8861) (-89.0564, 44.9546) (-88.2861, 45.0059) knots 0 0 0 1 2 2 2
  spline S158 degree 2 poles (-88.2861, 45.0059) (-87.7326, 45.0345) (-86.6198, 45.1029) (-85.6726, 45.16) (-84.9479, 45.2114) (-84.7767, 45.2285) knots 0 0 0 1 2 3 4 4 4
  spline S159 degree 2 poles (-84.7767, 45.2285) (-84.6112, 45.2399) (-84.2346, 45.2969) (-83.8523, 45.3483) (-83.5099, 45.3825) (-83.373, 45.3825) knots 0 0 0 1 2 3 4 4 4
  line L64 (-83.373, 45.3825) -> (-83.3559, 45.3825)
  spline S160 degree 2 poles (-83.3559, 45.3825) (-83.0991, 45.3825) (-82.7053, 45.3198) (-82.4486, 45.1657) (-82.3116, 44.9032) (-82.3116, 44.7035) knots 0 0 0 1 2 3 4 4 4
  spline S161 degree 2 poles (-82.3116, 44.7035) (-82.3116, 44.5494) (-82.4771, 44.1728) (-82.5798, 43.9103) knots 0 0 0 1 2 2 2
  spline S162 degree 2 poles (-82.5798, 43.9103) (-82.6768, 43.6592) (-82.8651, 43.237) (-83.0306, 42.8432) (-83.1675, 42.4495) (-83.2075, 42.2213) knots 0 0 0 1 2 3 4 4 4
  spline S163 degree 2 poles (-83.2075, 42.2213) (-83.2132, 42.1984) (-83.2417, 42.0044) (-83.276, 41.7362) (-83.3216, 41.4338) (-83.3616, 41.1656) (-83.3844, 40.9716) (-83.3844, 40.9431) knots 0 0 0 1 2 3 4 5 6 6 6
  spline S164 degree 2 poles (-83.3844, 40.9431) (-83.3844, 40.9202) (-83.3559, 40.8232) (-83.3559, 40.7947) knots 0 0 0 1 2 2 2
  spline S165 degree 2 poles (-83.3559, 40.7947) (-83.3559, 40.7148) (-83.4814, 40.5151) (-83.6069, 40.4124) knots 0 0 0 1 2 2 2
  spline S166 degree 2 poles (-83.6069, 40.4124) (-83.6754, 40.3553) (-83.9892, 40.2469) (-84.3659, 40.1499) (-84.7482, 40.0928) (-84.8851, 40.0928) knots 0 0 0 1 2 3 4 4 4
  spline S167 degree 2 poles (-84.8851, 40.0928) (-84.965, 40.0928) (-85.3017, 40.1214) (-85.6726, 40.1613) (-86.0036, 40.1898) (-86.072, 40.1898) knots 0 0 0 1 2 3 4 4 4
  spline S168 degree 2 poles (-86.072, 40.1898) (-86.2375, 40.1898) (-86.8081, 40.1955) (-87.1505, 40.1955) knots 0 0 0 1 2 2 2
  spline S169 degree 2 poles (-87.1505, 40.1955) (-87.7839, 40.1955) (-89.0735, 40.1499) (-89.7355, 40.0928) knots 0 0 0 1 2 2 2
  spline S170 degree 2 poles (-89.7355, 40.0928) (-90.0322, 40.07) (-90.5515, 39.9901) (-91.0479, 39.9159) (-91.5501, 39.8589) (-91.8354, 39.8589) knots 0 0 0 1 2 3 4 4 4
  spline S171 degree 2 poles (-91.8354, 39.8589) (-91.9723, 39.8589) (-92.2462, 39.9216) (-92.4688, 40.0244) (-92.6114, 40.1556) (-92.6114, 40.2241) knots 0 0 0 1 2 3 4 4 4
  spline S172 degree 2 poles (-96.3718, 40.652) (-96.3718, 40.7034) (-96.292, 40.9602) (-96.1322, 41.1485) knots 0 0 0 1 2 2 2
  spline S173 degree 2 poles (-96.1322, 41.1485) (-96.0124, 41.3026) (-95.8697, 41.5194) (-95.8526, 41.5765) knots 0 0 0 1 2 2 2
  spline S174 degree 2 poles (-95.8526, 41.5765) (-95.7213, 41.9873) (-95.4874, 42.9288) (-95.339, 43.4824) knots 0 0 0 1 2 2 2
  spline S175 degree 2 poles (-95.339, 43.4824) (-95.3048, 43.6307) (-95.2249, 43.9617) (-95.1678, 44.247) (-95.1336, 44.4695) (-95.1336, 44.5095) knots 0 0 0 1 2 3 4 4 4
  spline S176 degree 2 poles (-95.1336, 44.5095) (-95.1336, 44.538) (-95.1907, 44.6179) (-95.2591, 44.7035) (-95.3219, 44.7834) (-95.3219, 44.8119) knots 0 0 0 1 2 3 4 4 4
  spline S177 degree 2 poles (-95.3219, 44.8119) (-95.3219, 44.8975) (-95.1165, 45.063) (-94.8882, 45.1429) knots 0 0 0 1 2 2 2
  spline S178 degree 2 poles (-94.8882, 45.1429) (-94.6999, 45.2114) (-94.3233, 45.2798) (-94.135, 45.2855) knots 0 0 0 1 2 2 2
  spline S179 degree 2 poles (-94.135, 45.2855) (-93.7926, 45.2855) (-93.4103, 45.1143) (-93.2277, 44.8747) (-93.1992, 44.6179) (-93.1992, 44.5266) knots 0 0 0 1 2 3 4 4 4
  spline S180 degree 2 poles (-93.1992, 44.5266) (-93.1992, 44.3554) (-93.2334, 44.0416) (-93.2733, 43.8932) knots 0 0 0 1 2 2 2
  spline S181 degree 2 poles (-93.2733, 43.8932) (-93.3304, 43.6478) (-93.5472, 42.9916) (-93.6671, 42.6207) knots 0 0 0 1 2 2 2
  spline S182 degree 2 poles (-93.6671, 42.6207) (-93.6899, 42.5636) (-93.7812, 42.3126) (-93.9067, 41.9873) (-94.0437, 41.6221) (-94.1749, 41.2911) (-94.2719, 41.0287) (-94.2948, 40.9602) knots 0 0 0 1 2 3 4 5 6 6 6
  spline S183 degree 2 poles (-94.2948, 40.9602) (-94.3404, 40.8403) (-94.3804, 40.7148) (-94.426, 40.6007) (-94.4831, 40.4637) (-94.5344, 40.3439) knots 0 0 0 1 2 3 4 4 4
  line L65 (-94.5344, 40.3439) -> (-94.5287, 40.3496)
  spline S184 degree 2 poles (-94.5287, 40.3496) (-94.5401, 40.2925) (-94.6828, 40.1499) (-94.8939, 40.0244) (-95.1621, 39.9445) (-95.2877, 39.9445) knots 0 0 0 1 2 3 4 4 4
  spline S185 degree 2 poles (-95.2877, 39.9445) (-95.5958, 39.9445) (-96.0124, 40.0814) (-96.2634, 40.2868) (-96.3718, 40.5094) (-96.3718, 40.6007) knots 0 0 0 1 2 3 4 4 4
  line L66 (-96.3718, 40.6007) -> (-96.3718, 40.652)
  spline S186 degree 2 poles (-110.084, 45.023) (-110.0783, 45.12) (-109.8443, 45.2684) (-109.6389, 45.3255) knots 0 0 0 1 2 2 2
  spline S187 degree 2 poles (-109.6389, 45.3255) (-109.4906, 45.3654) (-109.1254, 45.4054) (-108.937, 45.4054) knots 0 0 0 1 2 2 2
  spline S188 degree 2 poles (-108.937, 45.4054) (-108.5034, 45.4054) (-107.6703, 45.2285) (-107.1852, 45.0687) knots 0 0 0 1 2 2 2
  spline S189 degree 2 poles (-107.1852, 45.0687) (-106.9456, 44.9888) (-106.2152, 44.7263) (-105.7358, 44.5437) knots 0 0 0 1 2 2 2
  spline S190 degree 2 poles (-105.7358, 44.5437) (-105.6217, 44.4981) (-104.9427, 44.2356) (-104.3834, 44.013) knots 0 0 0 1 2 2 2
  spline S191 degree 2 poles (-104.3834, 44.013) (-103.8642, 43.8076) (-103.2422, 43.5737) (-103.2023, 43.5622) knots 0 0 0 1 2 2 2
  spline S192 degree 2 poles (-103.2023, 43.5622) (-103.111, 43.5451) (-102.9455, 43.5394) (-102.7229, 43.5394) knots 0 0 0 1 2 2 2
  spline S193 degree 2 poles (-102.7229, 43.5394) (-102.6716, 43.5394) (-102.5746, 43.5394) (-102.4376, 43.5451) (-102.2151, 43.5508) (-102.0268, 43.5622) knots 0 0 0 1 2 3 4 4 4
  spline S194 degree 2 poles (-102.0268, 43.5622) (-101.5874, 43.4025) (-101.5874, 43.14) knots 0 0 0 1 1 1
  spline S195 degree 2 poles (-101.5874, 43.14) (-101.5874, 43.0087) (-101.8327, 42.8432) (-102.061, 42.8033) knots 0 0 0 1 2 2 2
  spline S196 degree 2 poles (-102.061, 42.8033) (-102.1181, 42.7976) (-102.1751, 42.7862) (-102.2436, 42.7862) (-102.3577, 42.7748) (-102.4661, 42.7691) knots 0 0 0 1 2 3 4 4 4
  spline S197 degree 2 poles (-102.4661, 42.7691) (-102.6716, 42.7691) (-103.0653, 42.7177) (-103.4305, 42.6435) (-103.7672, 42.5522) (-103.9269, 42.5123) knots 0 0 0 1 2 3 4 4 4
  spline S198 degree 2 poles (-103.9269, 42.5123) (-104.1609, 42.4552) (-104.6573, 42.3069) (-104.9084, 42.2213) knots 0 0 0 1 2 2 2
  spline S199 degree 2 poles (-104.9084, 42.2213) (-105.131, 42.1471) (-105.5589, 41.9645) (-105.7644, 41.8618) knots 0 0 0 1 2 2 2
  spline S200 degree 2 poles (-105.7644, 41.8618) (-105.9298, 41.7819) (-106.0839, 41.6107) (-106.0839, 41.5251) knots 0 0 0 1 2 2 2
  spline S201 degree 2 poles (-106.0839, 41.5251) (-106.0839, 41.3996) (-105.7644, 41.1713) (-105.285, 40.983) (-104.7144, 40.8461) (-104.4633, 40.8118) knots 0 0 0 1 2 3 4 4 4
  spline S202 degree 2 poles (-104.4633, 40.8118) (-103.9612, 40.7376) (-103.4819, 40.7376) knots 0 0 0 1 1 1
  spline S203 degree 2 poles (-103.4819, 40.7376) (-103.3392, 40.7376) (-102.9055, 40.7548) (-102.6373, 40.7662) knots 0 0 0 1 2 2 2
  spline S204 degree 2 poles (-102.6373, 40.7662) (-102.392, 40.7833) (-101.924, 40.8061) (-101.7072, 40.8232) knots 0 0 0 1 2 2 2
  spline S205 degree 2 poles (-101.7072, 40.8232) (-101.6045, 40.8346) (-101.4904, 40.8403) (-101.3762, 40.8518) (-101.2222, 40.8632) (-101.0966, 40.8803) knots 0 0 0 1 2 3 4 4 4
  spline S206 degree 2 poles (-101.0966, 40.8803) (-101.1537, 40.9488) (-101.2393, 41.0971) (-101.2735, 41.1884) knots 0 0 0 1 2 2 2
  spline S207 degree 2 poles (-101.2735, 41.1884) (-101.342, 41.3311) (-101.3762, 41.565) (-101.3762, 41.6563) knots 0 0 0 1 2 2 2
  spline S208 degree 2 poles (-101.3762, 41.6563) (-101.3762, 41.7648) (-101.3705, 41.9588) (-101.3534, 42.0558) knots 0 0 0 1 2 2 2
  spline S209 degree 2 poles (-101.3534, 42.0558) (-101.3306, 42.2441) (-101.2678, 42.4381) knots 0 0 0 1 1 1
  spline S210 degree 2 poles (-101.2678, 42.4381) (-101.2051, 42.6207) (-101.0966, 42.9231) knots 0 0 0 1 1 1
  spline S211 degree 2 poles (-101.0966, 42.9231) (-101.011, 43.1799) (-100.8912, 43.5679) (-100.857, 43.722) knots 0 0 0 1 2 2 2
  spline S212 degree 2 poles (-100.857, 43.722) (-100.8227, 43.8647) (-100.7828, 44.1386) (-100.7828, 44.2641) knots 0 0 0 1 2 2 2
  spline S213 degree 2 poles (-100.7828, 44.2641) (-100.7828, 44.3725) (-100.8284, 44.578) (-100.9197, 44.7663) (-101.0852, 44.9546) (-101.2108, 45.0573) knots 0 0 0 1 2 3 4 4 4
  spline S214 degree 2 poles (-101.2108, 45.0573) (-101.1366, 45.1143) (-100.914, 45.2114) (-100.663, 45.2912) (-100.4005, 45.3369) (-100.2863, 45.3369) knots 0 0 0 1 2 3 4 4 4
  spline S215 degree 2 poles (-100.2863, 45.3369) (-99.7043, 45.3369) (-99.4361, 45.2171) knots 0 0 0 1 1 1
  spline S216 degree 2 poles (-99.4361, 45.2171) (-99.1337, 45.0858) (-99.0709, 44.9146) knots 0 0 0 1 1 1
  spline S217 degree 2 poles (-99.0709, 44.9146) (-99.031, 44.829) (-99.0139, 44.6122) (-99.0139, 44.4752) knots 0 0 0 1 2 2 2
  spline S218 degree 2 poles (-99.0139, 44.4752) (-99.0139, 44.2755) (-99.0538, 44.0929) knots 0 0 0 1 1 1
  spline S219 degree 2 poles (-99.0538, 44.0929) (-99.0937, 43.9331) (-99.185, 43.6307) (-99.2421, 43.4824) knots 0 0 0 1 2 2 2
  spline S220 degree 2 poles (-99.2421, 43.4824) (-99.2763, 43.4196) (-99.322, 43.3055) (-99.3562, 43.1799) (-99.4019, 43.0316) (-99.4304, 42.9345) knots 0 0 0 1 2 3 4 4 4
  spline S221 degree 2 poles (-99.4304, 42.9345) (-99.5217, 42.6378) (-99.6415, 42.09) (-99.6415, 41.8618) knots 0 0 0 1 2 2 2
  spline S222 degree 2 poles (-99.6415, 41.8618) (-99.6415, 41.6906) (-99.6016, 41.314) (-99.5617, 41.1085) knots 0 0 0 1 2 2 2
  spline S223 degree 2 poles (-99.5617, 41.1085) (-99.3277, 41.1371) (-99.0139, 41.1713) (-98.9568, 41.1713) knots 0 0 0 1 2 2 2
  spline S224 degree 2 poles (-98.9568, 41.1713) (-98.5745, 41.1713) (-98.3177, 40.9887) (-98.3177, 40.8232) knots 0 0 0 1 2 2 2
  spline S225 degree 2 poles (-98.3177, 40.8232) (-98.3177, 40.6349) (-98.9682, 40.4751) knots 0 0 0 1 1 1
  spline S226 degree 2 poles (-98.9682, 40.4751) (-99.2193, 40.4124) (-99.7328, 40.3154) (-99.9839, 40.2754) knots 0 0 0 1 2 2 2
  spline S227 degree 2 poles (-99.9839, 40.2754) (-100.2635, 40.2298) (-101.0453, 40.1499) (-101.5132, 40.1157) knots 0 0 0 1 2 2 2
  spline S228 degree 2 poles (-101.5132, 40.1157) (-101.9583, 40.0814) (-102.7686, 40.0415) (-103.0824, 40.0415) knots 0 0 0 1 2 2 2
  spline S229 degree 2 poles (-103.0824, 40.0415) (-104.178, 40.0415) (-105.1937, 40.1727) knots 0 0 0 1 1 1
  spline S230 degree 2 poles (-105.1937, 40.1727) (-105.7301, 40.2412) (-106.626, 40.4694) (-106.9741, 40.6349) knots 0 0 0 1 2 2 2
  spline S231 degree 2 poles (-106.9741, 40.6349) (-107.7559, 40.983) (-107.7559, 41.5365) knots 0 0 0 1 1 1
  spline S232 degree 2 poles (-107.7559, 41.5365) (-107.7559, 41.896) (-107.2023, 42.2498) knots 0 0 0 1 1 1
  spline S233 degree 2 poles (-107.2023, 42.2498) (-106.7344, 42.5351) (-105.519, 42.9631) (-104.7943, 43.1628) knots 0 0 0 1 2 2 2
  spline S234 degree 2 poles (-104.7943, 43.1628) (-105.0226, 43.2484) (-105.4848, 43.4139) (-105.753, 43.4995) knots 0 0 0 1 2 2 2
  spline S235 degree 2 poles (-105.753, 43.4995) (-106.1467, 43.6364) (-106.8314, 43.8818) (-107.1339, 43.9902) knots 0 0 0 1 2 2 2
  spline S236 degree 2 poles (-107.1339, 43.9902) (-107.4363, 44.0929) (-108.1667, 44.344) (-108.6061, 44.4981) knots 0 0 0 1 2 2 2
  spline S237 degree 2 poles (-108.6061, 44.4981) (-109.0226, 44.635) (-109.7245, 44.8633) (-109.9528, 44.9374) knots 0 0 0 1 2 2 2
  line L67 (-109.9528, 44.9374) -> (-110.084, 45.023)
  spline S238 degree 2 poles (-120.6007, 43.294) (-120.6007, 43.4652) (-120.4694, 43.7791) (-120.2126, 44.0872) (-119.8189, 44.3954) (-119.5621, 44.5665) knots 0 0 0 1 2 3 4 4 4
  spline S239 degree 2 poles (-119.5621, 44.5665) (-119.4081, 44.6578) (-119.0942, 44.8347) (-118.7918, 44.9888) (-118.5008, 45.1086) (-118.3866, 45.1486) knots 0 0 0 1 2 3 4 4 4
  spline S240 degree 2 poles (-118.3866, 45.1486) (-118.1584, 45.2285) (-117.4223, 45.394) (-116.9601, 45.4681) knots 0 0 0 1 2 2 2
  spline S241 degree 2 poles (-116.9601, 45.4681) (-116.515, 45.5366) (-115.659, 45.6108) (-115.2938, 45.6108) knots 0 0 0 1 2 2 2
  spline S242 degree 2 poles (-115.2938, 45.6108) (-114.9172, 45.6108) (-114.3181, 45.5423) (-113.9015, 45.3997) (-113.679, 45.1828) (-113.679, 45.0287) knots 0 0 0 1 2 3 4 4 4
  spline S243 degree 2 poles (-113.679, 45.0287) (-113.679, 44.9317) (-113.8501, 44.772) (-114.1469, 44.6635) (-114.5463, 44.6008) (-114.7689, 44.6008) knots 0 0 0 1 2 3 4 4 4
  spline S244 degree 2 poles (-114.7689, 44.6008) (-114.9058, 44.6008) (-115.0998, 44.6122) (-115.271, 44.635) (-115.4365, 44.6693) (-115.5449, 44.6921) knots 0 0 0 1 2 3 4 4 4
  spline S245 degree 2 poles (-115.5449, 44.6921) (-115.893, 44.772) (-116.0813, 44.772) knots 0 0 0 1 1 1
  spline S246 degree 2 poles (-116.0813, 44.772) (-116.1726, 44.772) (-116.4979, 44.7377) (-116.8459, 44.6864) (-117.1598, 44.6179) (-117.2454, 44.5894) knots 0 0 0 1 2 3 4 4 4
  spline S247 degree 2 poles (-117.2454, 44.5894) (-117.5307, 44.4924) (-118.107, 44.207) (-118.5749, 43.8818) (-118.8717, 43.5394) (-118.8717, 43.3853) knots 0 0 0 1 2 3 4 4 4
  spline S248 degree 2 poles (-118.8717, 43.3853) (-118.8717, 43.2598) (-118.6434, 43.0601) (-118.301, 42.9003) (-117.8674, 42.7862) (-117.4622, 42.712) (-117.1198, 42.6778) (-117.0228, 42.6778) knots 0 0 0 1 2 3 4 5 6 6 6
  spline S249 degree 2 poles (-117.0228, 42.6778) (-116.766, 42.6778) (-116.4066, 42.6949) (-116.1212, 42.7291) (-115.8702, 42.7805) (-115.7275, 42.809) knots 0 0 0 1 2 3 4 4 4
  spline S250 degree 2 poles (-115.7275, 42.809) (-115.5563, 42.849) (-115.311, 42.8832) (-115.1797, 42.8832) knots 0 0 0 1 2 2 2
  spline S251 degree 2 poles (-115.1797, 42.8832) (-114.9971, 42.8832) (-114.6947, 42.8261) (-114.4892, 42.7234) (-114.3694, 42.5922) (-114.3694, 42.5294) knots 0 0 0 1 2 3 4 4 4
  spline S252 degree 2 poles (-114.3694, 42.5294) (-114.3694, 42.4096) (-114.5235, 42.2156) (-114.7803, 42.0729) (-115.1112, 41.9873) (-115.2938, 41.9645) knots 0 0 0 1 2 3 4 4 4
  spline S253 degree 2 poles (-115.2938, 41.9645) (-115.3965, 41.9588) (-115.6476, 41.9474) (-115.8873, 41.9474) (-116.0642, 41.9474) (-116.087, 41.9417) knots 0 0 0 1 2 3 4 4 4
  spline S254 degree 2 poles (-116.087, 41.9417) (-116.2468, 41.896) (-116.6862, 41.7534) (-117.1598, 41.5765) (-117.6391, 41.3824) (-118.0214, 41.1884) (-118.2497, 41.0172) (-118.2497, 40.9488) knots 0 0 0 1 2 3 4 5 6 6 6
  spline S255 degree 2 poles (-118.2497, 40.9488) (-118.2497, 40.8175) (-117.7646, 40.6863) (-117.2168, 40.6863) knots 0 0 0 1 2 2 2
  spline S256 degree 2 poles (-117.2168, 40.6863) (-116.7889, 40.6863) (-115.6819, 40.7719) (-115.1569, 40.8518) knots 0 0 0 1 2 2 2
  spline S257 degree 2 poles (-115.1569, 40.8518) (-114.9343, 40.8917) (-114.4892, 40.9887) (-114.0898, 41.1085) (-113.7703, 41.2341) (-113.6733, 41.3026) knots 0 0 0 1 2 3 4 4 4
  spline S258 degree 2 poles (-113.6733, 41.3026) (-113.6504, 41.314) (-113.6219, 41.4281) (-113.6048, 41.6449) (-113.5877, 41.9759) (-113.5648, 42.2099) knots 0 0 0 1 2 3 4 4 4
  spline S259 degree 2 poles (-113.5648, 42.2099) (-113.5477, 42.3639) (-113.5306, 42.5579) (-113.4964, 42.7291) (-113.4564, 42.9174) (-113.4222, 43.0658) knots 0 0 0 1 2 3 4 4 4
  spline S260 degree 2 poles (-113.4222, 43.0658) (-113.3594, 43.2712) (-113.2681, 43.6478) (-113.2681, 43.7848) knots 0 0 0 1 2 2 2
  line L68 (-113.2681, 43.7848) -> (-113.2681, 44.4467)
  spline S261 degree 2 poles (-113.2681, 44.4467) (-113.2681, 44.8005) (-112.7374, 45.1315) (-112.2182, 45.1315) knots 0 0 0 1 2 2 2
  spline S262 degree 2 poles (-112.2182, 45.1315) (-111.9443, 45.1315) (-111.5791, 45.0287) (-111.3736, 44.829) (-111.2937, 44.5266) (-111.2937, 44.3269) knots 0 0 0 1 2 3 4 4 4
  spline S263 degree 2 poles (-111.2937, 44.3269) (-111.2937, 44.3212) (-111.3394, 44.1671) (-111.4022, 43.9331) (-111.482, 43.6535) (-111.5505, 43.4025) (-111.6019, 43.2027) (-111.6133, 43.1685) knots 0 0 0 1 2 3 4 5 6 6 6
  spline S264 degree 2 poles (-111.6133, 43.1685) (-111.619, 43.1571) (-111.6532, 42.9631) (-111.7103, 42.6949) (-111.7674, 42.3867) (-111.8244, 42.1128) (-111.8701, 41.9188) (-111.8701, 41.896) knots 0 0 0 1 2 3 4 5 6 6 6
  spline S265 degree 2 poles (-111.8701, 41.896) (-111.9328, 41.6221) (-111.9328, 41.565) knots 0 0 0 1 1 1
  spline S266 degree 2 poles (-111.9328, 41.565) (-111.9328, 41.5251) (-111.9043, 41.4281) (-111.8701, 41.3197) (-111.8415, 41.2398) (-111.8415, 41.2227) knots 0 0 0 1 2 3 4 4 4
  spline S267 degree 2 poles (-111.8415, 41.2227) (-111.8415, 41.0857) (-111.9443, 40.8403) (-112.0584, 40.7376) knots 0 0 0 1 2 2 2
  spline S268 degree 2 poles (-112.0584, 40.7376) (-112.3437, 40.458) (-112.6747, 40.4352) knots 0 0 0 1 1 1
  spline S269 degree 2 poles (-112.6747, 40.4352) (-112.8858, 40.4238) (-113.2966, 40.3667) (-113.4792, 40.3382) knots 0 0 0 1 2 2 2
  spline S270 degree 2 poles (-113.4792, 40.3382) (-114.3808, 40.1955) (-115.4251, 40.0129) (-115.5906, 39.9901) knots 0 0 0 1 2 2 2
  spline S271 degree 2 poles (-115.5906, 39.9901) (-115.8074, 39.9559) (-116.2525, 39.9102) (-116.7546, 39.8874) (-117.3538, 39.876) (-117.7304, 39.876) knots 0 0 0 1 2 3 4 4 4
  spline S272 degree 2 poles (-117.7304, 39.876) (-117.9587, 39.876) (-118.5179, 39.9559) (-119.0371, 40.0928) (-119.4765, 40.2754) (-119.5907, 40.3781) knots 0 0 0 1 2 3 4 4 4
  spline S273 degree 2 poles (-119.5907, 40.3781) (-119.642, 40.4238) (-119.7333, 40.555) (-119.8132, 40.6977) (-119.8588, 40.8403) (-119.8588, 40.8917) knots 0 0 0 1 2 3 4 4 4
  spline S274 degree 2 poles (-119.8588, 40.8917) (-119.8588, 41.1656) (-118.9972, 41.7419) (-118.1755, 42.0843) knots 0 0 0 1 2 2 2
  spline S275 degree 2 poles (-118.1755, 42.0843) (-118.6662, 42.1642) (-119.545, 42.4153) (-120.2126, 42.7405) (-120.6007, 43.1057) (-120.6007, 43.294) knots 0 0 0 1 2 3 4 4 4
  line L69 (-152.4169, 57.2192) -> (-147.9334, 57.2192)
  line L70 (-147.9334, 57.2192) -> (-147.9334, 56.2256)
  spline S276 degree 2 poles (-147.9334, 56.2256) (-148.5019, 55.7708) (-149.4114, 54.97) (-149.7525, 54.6091) knots 0 0 0 1 2 2 2
  spline S277 degree 2 poles (-149.7525, 54.6091) (-150.2023, 54.1395) (-150.6028, 53.4227) (-150.6028, 53.047) knots 0 0 0 1 2 2 2
  spline S278 degree 2 poles (-150.6028, 53.047) (-150.6028, 52.6219) (-150.0936, 52.1671) (-149.6388, 52.1671) knots 0 0 0 1 2 2 2
  spline S279 degree 2 poles (-149.6388, 52.1671) (-149.4065, 52.1671) (-148.9912, 52.2808) (-148.7787, 52.3698) knots 0 0 0 1 2 2 2
  spline S280 degree 2 poles (-148.7787, 52.3698) (-148.5711, 52.4637) (-148.2745, 52.6615) (-148.2003, 52.7109) knots 0 0 0 1 2 2 2
  line L71 (-148.2003, 52.7109) -> (-148.0817, 52.7109)
  line L72 (-148.0817, 52.7109) -> (-148.0817, 51.3811)
  spline S281 degree 2 poles (-148.0817, 51.3811) (-148.3387, 51.2576) (-149.4361, 51.0005) (-149.9453, 51.0005) knots 0 0 0 1 2 2 2
  spline S282 degree 2 poles (-149.9453, 51.0005) (-151.0328, 51.0005) (-152.15, 51.9694) (-152.15, 52.8444) knots 0 0 0 1 2 2 2
  spline S283 degree 2 poles (-152.15, 52.8444) (-152.15, 53.3832) (-151.6408, 54.4213) (-151.0526, 55.0145) knots 0 0 0 1 2 2 2
  spline S284 degree 2 poles (-151.0526, 55.0145) (-150.6818, 55.3803) (-149.9848, 55.9487) (-149.8316, 56.0674) knots 0 0 0 1 2 2 2
  line L73 (-149.8316, 56.0674) -> (-152.4169, 56.0674)
  line L74 (-152.4169, 56.0674) -> (-152.4169, 57.2192)
  spline S285 degree 2 poles (-157.6815, 54.1692) (-157.6815, 54.9601) (-157.4294, 56.1465) (-157.1476, 56.5469) knots 0 0 0 1 2 2 2
  spline S286 degree 2 poles (-157.1476, 56.5469) (-156.8708, 56.9423) (-155.9761, 57.3477) (-155.3335, 57.3477) knots 0 0 0 1 2 2 2
  spline S287 degree 2 poles (-155.3335, 57.3477) (-154.6859, 57.3477) (-153.7961, 56.9423) (-153.5143, 56.537) knots 0 0 0 1 2 2 2
  spline S288 degree 2 poles (-153.5143, 56.537) (-153.2326, 56.1366) (-152.9805, 54.9601) (-152.9805, 54.1692) knots 0 0 0 1 2 2 2
  spline S289 degree 2 poles (-152.9805, 54.1692) (-152.9805, 53.3585) (-153.2326, 52.2116) (-153.5193, 51.7964) knots 0 0 0 1 2 2 2
  spline S290 degree 2 poles (-153.5193, 51.7964) (-153.806, 51.391) (-154.7106, 50.9956) (-155.3335, 50.9956) knots 0 0 0 1 2 2 2
  spline S291 degree 2 poles (-155.3335, 50.9956) (-155.9909, 50.9956) (-156.8708, 51.4108) (-157.1526, 51.8211) knots 0 0 0 1 2 2 2
  spline S292 degree 2 poles (-157.1526, 51.8211) (-157.4294, 52.2215) (-157.6815, 53.4029) (-157.6815, 54.1692) knots 0 0 0 1 2 2 2
  spline S293 degree 2 poles (-156.1442, 54.1692) (-156.1442, 53.0371) (-155.7734, 52.1226) (-155.3335, 52.1226) knots 0 0 0 1 2 2 2
  spline S294 degree 2 poles (-155.3335, 52.1226) (-154.8935, 52.1226) (-154.5178, 53.0371) (-154.5178, 54.1741) knots 0 0 0 1 2 2 2
  spline S295 degree 2 poles (-154.5178, 54.1741) (-154.5178, 55.2913) (-154.8935, 56.2206) (-155.3335, 56.2206) knots 0 0 0 1 2 2 2
  spline S296 degree 2 poles (-155.3335, 56.2206) (-155.7685, 56.2206) (-156.1442, 55.2913) (-156.1442, 54.1692) knots 0 0 0 1 2 2 2
  line L75 (-162.8324, 57.2192) -> (-158.8036, 57.2192)
  line L76 (-158.8036, 57.2192) -> (-158.8036, 56.1563)
  line L77 (-158.8036, 56.1563) -> (-160.0889, 56.1563)
  line L78 (-160.0889, 56.1563) -> (-160.0889, 52.9284)
  line L79 (-160.0889, 52.9284) -> (-158.8036, 52.9284)
  line L80 (-158.8036, 52.9284) -> (-158.8036, 51.9348)
  spline S297 degree 2 poles (-158.8036, 51.9348) (-159.0854, 51.9348) (-159.644, 51.8606) (-159.8121, 51.7816) knots 0 0 0 1 2 2 2